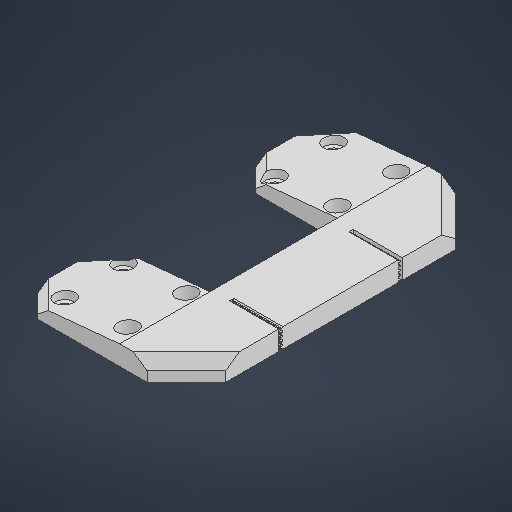
# Autodesk Inventor part: X-Base Cover
Saved by Autodesk Inventor 2025.1 (Build 291241000, 241)
## iProperties
Created: 2025-02-18
Part Number: X-Base Cover
Material: Generic
Document SubType Name: Modeling
Designer: jerem
Density: 1 g/cm^3
Appearance: Default
Author: jerem
## iProperties of the stored document X Axis Base Plate Accurate_3DPrint.ipt
Created: 2025-02-18
Part Number: X Axis Base Plate Accurate_3DPrint
Material: Generic
Document SubType Name: Modeling
Designer: jerem
Density: 1 g/cm^3
Appearance: Default
Author: jerem
Autodesk Inventor part; units mm, degrees
ref_plane "YZ Plane" through (0, 0, 0) normal (1, 0, 0) x (0, 1, 0)
ref_plane "XZ Plane" through (0, 0, 0) normal (0, 1, 0) x (-1, 0, 0)
ref_plane "XY Plane" through (0, 0, 0) normal (0, 0, 1) x (1, 0, 0)
sketch "Sketch1" plane through (0, 0, 0) normal (0, 1, 0) x (-1, 0, 0)
  line L0 (0, 0) -> (-86, 0)
  line L1 (-86, 0) -> (-86, -157)
  line L2 (-86, -157) -> (0, -157)
  line L3 (0, -157) -> (0, 0)
  line L4 (-14, -40) -> (-46, -40) construction
  line L5 (-46, -40) -> (-46, -10) construction
  line L6 (-46, -10) -> (-14, -10) construction
  line L7 (-14, -10) -> (-14, -40) construction
  line L8 (-14, -147) -> (-46, -147) construction
  line L9 (-46, -147) -> (-46, -117) construction
  line L10 (-46, -117) -> (-14, -117) construction
  line L11 (-14, -117) -> (-14, -147) construction
  line L12 (0, -46) -> (-52, -46)
  line L13 (-52, -46) -> (-52, -111)
  line L14 (-52, -111) -> (0, -111)
  dimension "d0" = 86
  dimension "d1" = 157
  dimension "d2" = 32
  dimension "d3" = 30
  dimension "d4" = 14
  dimension "d5" = 10
  dimension "d6" = 32
  dimension "d7" = 30
  dimension "d8" = 10
  dimension "d9" = 14
  dimension "d36" = 52
  dimension "d37" = 46
  dimension "d38" = 46
  dimension "d39" = 65
  constraints: 30 end point, 6 parallel, 5 perpendicular, 4 coincident, 4 horizontal, 2 point on line
  measures "d0" distance of L2.end L1.end
  measures "d1" distance of L1.end L0.end
  measures "d2" distance of L4.start L4.end
  measures "d3" distance of L6.end L4.start
  measures "d4" distance between parallel lines of L3 L7
  measures "d5" distance between parallel lines of L0 L6
  measures "d6" distance of L8.start L8.end
  measures "d7" distance of L10.end L8.start
  measures "d8" distance between parallel lines of L2 L8
  measures "d9" distance between parallel lines of L3 L11
  measures "d36" distance of L12.start L12.end
  measures "d37" distance between parallel lines of L0 L12
  measures "d38" distance between parallel lines of L2 L14
  measures "d39" distance of L12.end L13.end
extrude "Extrusion1" add sketch "Sketch1" along normal blind 10 contours L3 L12 L13 L14 L2 L1 L0
sketch "Sketch2" plane through (86, 0, 0) normal (1, 0, 0) x (0, 0, -1)
  line L0 (0, 0) -> (157, 0) projected
  line L1 (157, 0) -> (157, 10) projected
  line L2 (0, 10) -> (157, 10) projected
  line L3 (0, 0) -> (0, 10) projected
  line L4 (47, 10) -> (47, 0)
  line L5 (110, 10) -> (110, 0)
  arc A0 (109, 1.1286) -> (108.7921, 1.375) centre (108.75, 1.1286) ccw
  arc A1 (108.7921, 0.625) -> (109, 0.8714) centre (108.75, 0.8714) ccw
  line L6 (109, 0.8714) -> (109, 1.1286)
  line L7 (107.85, 0) -> (106.3073, 0)
  arc A2 (107.85, 2) -> (108.3073, 1.4579) centre (108.4, 2) ccw
  line L8 (108.3073, 1.4579) -> (108.7921, 1.375)
  line L9 (108.7921, 0.625) -> (108.3073, 0.5421)
  arc A3 (108.3073, 0.5421) -> (107.85, 0) centre (108.4, 0) ccw
  line L10 (107.85, 2) -> (106.3073, 2)
  line L11 (106.3073, 2) -> (106.3073, 0)
  line L12 (108.3073, 1.4579) -> (108.3073, 0.5421) construction
  line L13 (108.3073, 1) -> (109, 1) construction
  line L14 (108.3073, 1) -> (106.3073, 1) construction
  line L15 (78.5, 10) -> (78.5, 0) construction
  line L16 (49.15, 2) -> (50.6927, 2)
  line L17 (50.6927, 2) -> (50.6927, 0)
  line L18 (49.15, 0) -> (50.6927, 0)
  arc A4 (48.2079, 1.375) -> (48, 1.1286) centre (48.25, 1.1286) ccw
  arc A5 (48, 0.8714) -> (48.2079, 0.625) centre (48.25, 0.8714) ccw
  line L19 (48.2079, 0.625) -> (48.6927, 0.5421)
  arc A6 (49.15, 0) -> (48.6927, 0.5421) centre (48.6, 0) ccw
  line L20 (48, 0.8714) -> (48, 1.1286)
  line L21 (48.6927, 1.4579) -> (48.2079, 1.375)
  arc A7 (48.6927, 1.4579) -> (49.15, 2) centre (48.6, 2) ccw
  line L22 (48.6927, 1.4579) -> (48.6927, 0.5421) construction
  line L23 (48.6927, 1) -> (48, 1) construction
  line L24 (48.6927, 1) -> (50.6927, 1) construction
  line L25 (49.15, 2) -> (47, 2)
  line L26 (107.85, 2) -> (110, 2)
  point P0 (49.15, 0)
  dimension "d40" = 47
  dimension "d41" = 47
  dimension "d49" = 0.2571
  dimension "d50" = 0.6927
  dimension "d51" = 2
  dimension "d52" = 0.25
  dimension "d53" = 1
  dimension "d60" = 1
  dimension "d65" = 0.55
  dimension "d66" = 0.9157
  constraints: 46 end point, 18 point on circle, 17 symmetric about line, 8 centre point, 7 point on line, 6 perpendicular, 6 tangent, 5 midpoint, 2 equal length, 2 equal radius, 1 horizontal, 1 line through centre, 1 parallel, 1 vertical, 4 other
  measures "d40" distance between parallel lines of L3 L4
  measures "d41" distance between parallel lines of L1 L5
  measures "d49" distance of L6.start L6.end
  measures "d50" distance of L13.start L13.end
  measures "d51" distance of L13.start L14.end
  measures "d52" radius of A1
  measures "d53" distance between parallel lines of L5 L6
  measures "d60" distance between parallel lines of L4 L20
  measures "d65" radius of A2
  measures "d66" distance of L8.start L9.end
extrude "Extrusion2" cut sketch "Sketch2" against normal blind 25 contours L4 L25 A7 L21 A4 L20 A5 L19 A6 L0 | L5 L0 A3 L9 A1 L6 A0 L8 A2 L26
pattern_linear "Rectangular Pattern1" count 5 spacing 2 along (0, 1, 0) of "Extrusion2"
sketch "Sketch3" plane through (0, 10, 0) normal (0, 1, 0) x (1, 0, 0)
  line L0 (61, 49.15) -> (86, 49.15) projected
  line L1 (86, 49.15) -> (86, 107.85) projected
  line L2 (86, 107.85) -> (61, 107.85) projected
  line L3 (61, 107.85) -> (61, 110) projected
  line L4 (61, 110) -> (86, 110) projected
  line L5 (86, 110) -> (86, 157) projected
  line L6 (86, 157) -> (0, 157) projected
  line L7 (0, 157) -> (0, 111) projected
  line L8 (0, 0) -> (86, 0) projected
  line L9 (86, 0) -> (86, 47) projected
  line L10 (86, 47) -> (61, 47) projected
  line L11 (61, 47) -> (61, 49.15) projected
  line L12 (46, 117) -> (14, 117) construction
  line L13 (14, 117) -> (14, 147) construction
  line L14 (14, 147) -> (46, 147) construction
  line L15 (46, 147) -> (46, 117) construction
  line L16 (46, 10) -> (14, 10) construction
  line L17 (14, 10) -> (14, 40) construction
  line L18 (14, 40) -> (46, 40) construction
  line L19 (46, 40) -> (46, 10) construction
  line L20 (0, 111) -> (52, 111) projected
  line L21 (52, 111) -> (52, 46) projected
  line L22 (52, 46) -> (0, 46) projected
  line L23 (0, 46) -> (0, 0) projected
  dimension "d72" = 32
  dimension "d73" = 30
  dimension "d74" = 32
  dimension "d75" = 30
  dimension "d76" = 10
  dimension "d77" = 10
  dimension "d78" = 14
  dimension "d79" = 14
  constraints: 16 end point, 4 coincident, 4 parallel, 2 horizontal, 2 perpendicular
  measures "d72" distance of L12.start L13.start
  measures "d73" distance of L15.start L12.start
  measures "d74" distance of L19.end L17.start
  measures "d75" distance of L18.end L19.end
  measures "d76" distance between parallel lines of L6 L14
  measures "d77" distance between parallel lines of L8 L16
  measures "d78" distance between parallel lines of L7 L17
  measures "d79" distance between parallel lines of L7 L13
hole "Hole3" at (14, 10, -147) at (46, 10, -117) at (46, 10, -147) at (14, 10, -117) at (14, 10, -40) at (46, 10, -10) at (14, 10, -10) at (46, 10, -40) direction (0, -1, 0) diameter 5.6 end through all counterbore diameter 10 counterbore depth 8
chamfer "Chamfer1" distance 20 angle 45 2 edges at (86, 5, 0) (86, 5, -157)
chamfer "Chamfer2" distance 10 angle 45 4 edges at (0, 5, -157) (0, 5, -111) (0, 5, -46) (0, 5, 0)
chamfer "Chamfer3" distance 5 angle 45 2 edges at (76, 10, -10) (76, 10, -147)
chamfer "Chamfer4" distance 52 distance2 5 2 edges at (0, 10, -134) (0, 10, -23)
chamfer "Chamfer5" distance 4 angle 45 4 edges at (5, 5.4808, -116) (5, 5.4808, -152) (5, 5.4808, -41) (5, 5.4808, -5)
equation "\"d6\" = d2"
equation "\"d7\" = d3"
equation "\"d38\" = d37"
body "Solid1"
